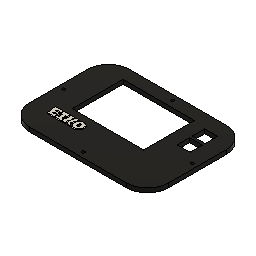
top plate (Autodesk Fusion 360 design; units mm, degrees)
part number: 2026-08-25-02-54-07-841
Autodesk Fusion 360 part; units mm, degrees
note: some values were not read from the file. Chosen so that the rebuilt part matches the saved one: which bodies a step acts on.
sketch "Sketch1" plane through (0, 0, 0) normal (0, 1, 0) x (1, 0, 0)
  line L0 (-1.5154, 62.1887) -> (-1.5154, -12.2213)
  line L1 (-112.7654, -12.2213) -> (-112.7654, 62.1887)
  line L2 (-112.7654, 62.1887) -> (-1.5154, 62.1887)
  line L3 (-1.5154, -12.2213) -> (-112.7654, -12.2213)
  line L4 (-122.7654, 72.1887) -> (8.4846, 72.1887)
  line L5 (-122.7654, -22.2213) -> (-122.7654, 72.1887)
  line L6 (8.4846, 72.1887) -> (8.4846, -22.2213)
  line L7 (8.4846, -22.2213) -> (-122.7654, -22.2213)
  circle A0 centre (-117.7654, 24.9837) radius 1.35
  circle A1 centre (-57.1404, 67.1887) radius 1.35
  circle A2 centre (3.4846, 24.9837) radius 1.35
  circle A3 centre (-57.1404, -17.2213) radius 1.35
sketch "Sketch2" plane through (0, 0, 0) normal (0, 1, 0) x (1, 0, 0)
  line L0 (-106.5854, 60.9687) -> (-21.5854, 60.9687)
  line L1 (-21.5854, 60.9687) -> (-21.5854, 12.9687)
  line L2 (-21.5854, 12.9687) -> (-106.5854, 12.9687)
  line L3 (-106.5854, 12.9687) -> (-106.5854, 60.9687)
  line L4 (-106.5854, 60.9687) -> (-21.5854, 60.9687)
  line L5 (-21.5854, 60.9687) -> (-21.5854, 12.9687)
  line L6 (-21.5854, 12.9687) -> (-106.5854, 12.9687)
  line L7 (-106.5854, 12.9687) -> (-106.5854, 60.9687)
  line L8 (-18.6954, 59) -> (-6.4954, 59)
  line L9 (-6.4954, 59) -> (-6.4954, 47.3)
  line L10 (-6.4954, 47.3) -> (-18.6954, 47.3)
  line L11 (-18.6954, 47.3) -> (-18.6954, 59)
  line L12 (-18.6954, 44.63) -> (-6.4954, 44.63)
  line L13 (-6.4954, 44.63) -> (-6.4954, 32.93)
  line L14 (-6.4954, 32.93) -> (-18.6954, 32.93)
  line L15 (-18.6954, 32.93) -> (-18.6954, 44.63)
  line L16 (-97.8354, 60.9687) -> (-30.3354, 60.9687)
  line L17 (-30.3354, 60.9687) -> (-30.3354, 12.9687)
  line L18 (-30.3354, 12.9687) -> (-97.8354, 12.9687)
  line L19 (-97.8354, 12.9687) -> (-97.8354, 60.9687)
  dimension "d5" = 85
  dimension "d6" = 48
  dimension "d11" = 12.2
  dimension "d12" = 11.7
  dimension "d13" = 2.89
  dimension "d14" = 12.2
  dimension "d15" = 11.7
  dimension "d16" = 2.67
  dimension "d17" = 2.89
  dimension "d28" = 67.5
  dimension "d29" = 8.75
  constraint horizontal L0
  constraint vertical L1
  constraint horizontal L2
  constraint vertical L3
  constraint horizontal L4
  constraint vertical L5
  constraint horizontal L6
  constraint vertical L7
  constraint horizontal L8
  constraint vertical L9
  constraint horizontal L10
  constraint vertical L11
  constraint horizontal L12
  constraint vertical L13
  constraint horizontal L14
  constraint vertical L15
  constraint horizontal L16
  constraint vertical L17
  constraint horizontal L18
  constraint vertical L19
  constraint coincident L4 L16.start
  measures "d5" distance of L0.start L0.end
  measures "d6" distance of L0 L2
  measures "d11" distance of L8.start L8.end
  measures "d12" distance of L8.start L10.end
  measures "d13" distance of L5 L11
  measures "d14" distance of L12.start L12.end
  measures "d15" distance of L12.start L14.end
  measures "d16" distance of L10 L12
  measures "d17" distance of L5 L15
  measures "d28" distance of L16.start L16.end
  measures "d29" distance of L7 L19
extrude "Extrude1" add sketch "Sketch1" along normal blind 4 contours L0 L1 L2 L3 | L4 L5 L6 L7 makes body 1
sketch "Sketch3" plane through (0, 4, 0) normal (0, 1, 0) x (-1, 0, 0)
  circle A0 centre (117.7654, -24.9837) radius 1.35
  circle A1 centre (57.1404, 17.2213) radius 1.35
  circle A2 centre (-3.4846, -24.9837) radius 1.35
  circle A3 centre (57.1404, -67.1887) radius 1.35
  line L0 (-8.4846, 22.2213) -> (-8.4846, -72.1887)
  line L1 (-8.4846, -72.1887) -> (122.7654, -72.1887)
  line L2 (122.7654, -72.1887) -> (122.7654, 22.2213)
  line L3 (122.7654, 22.2213) -> (-8.4846, 22.2213)
extrude "Extrude2" cut sketch "Sketch2" along normal blind 10 bodies 1
fillet "Fillet1" radius 20 4 edges at (-122.7654, 2, 22.2213) (8.4846, 2, 22.2213) (8.4846, 2, -72.1887) (-122.7654, 2, -72.1887) on bodies 1
sketch "Sketch4" plane through (0, 4, 0) normal (0, 1, 0) x (-1, 0, 0)
sketch "Sketch5" plane through (0, 4, 0) normal (0, 1, 0) x (-1, 0, 0)
  line L0 (99.062, -5.8308) -> (106.6622, -5.8308)
  line L1 (106.6622, -5.8308) -> (105.2136, 2.8806)
  line L2 (105.2136, 2.8806) -> (98.804, 2.9004)
  line L3 (98.804, 2.9004) -> (98.804, -0.1357)
  line L4 (98.804, -0.1357) -> (102.8919, 0.8168)
  line L5 (102.8919, 0.8168) -> (102.8919, -0.5325)
  line L6 (102.8919, -0.5325) -> (98.9231, -0.5325)
  line L7 (98.9231, -0.5325) -> (99.062, -2.6955)
  line L8 (99.062, -2.6955) -> (102.8919, -2.4177)
  line L9 (102.8919, -2.4177) -> (102.6934, -3.8068)
  line L10 (102.6934, -3.8068) -> (98.804, -3.1519)
  line L11 (98.804, -3.1519) -> (99.062, -5.8308)
  line L12 (98.2484, 0.539) -> (98.2484, 2.9798)
  line L13 (98.2484, 2.9798) -> (92.5334, 2.8806)
  line L14 (92.5334, 2.8806) -> (92.6922, 0.539)
  line L15 (92.6922, 0.539) -> (94.0217, 0.4795)
  line L16 (94.0217, 0.4795) -> (94.0217, -2.9535)
  line L17 (94.0217, -2.9535) -> (92.5533, -3.1916)
  line L18 (92.5533, -3.1916) -> (92.6922, -6.0491)
  line L19 (92.6922, -6.0491) -> (98.4667, -6.0491)
  line L20 (98.4667, -6.0491) -> (98.4667, -2.5963)
  line L21 (98.4667, -2.5963) -> (96.8792, -2.8543)
  line L22 (96.8792, -2.8543) -> (96.7006, 0.539)
  line L23 (96.7006, 0.539) -> (98.2484, 0.539)
  line L24 (91.819, -6.0094) -> (91.5809, -0.5921)
  line L25 (91.5809, -0.5921) -> (92.0373, -0.5921)
  line L26 (92.0373, -0.5921) -> (92.0373, 2.7417)
  line L27 (92.0373, 2.7417) -> (89.0806, 2.7417)
  line L28 (89.0806, 2.7417) -> (89.0806, -0.5921)
  line L29 (89.0806, -0.5921) -> (86.739, 2.7417)
  line L30 (86.739, 2.7417) -> (84.199, 2.7417)
  line L31 (84.199, 2.7417) -> (86.4612, -0.5921)
  line L32 (86.4612, -0.5921) -> (85.8262, -0.5921)
  line L33 (85.8262, -0.5921) -> (83.6633, -6.0094)
  line L34 (83.6633, -6.0094) -> (87.1161, -6.0094)
  line L35 (87.1161, -6.0094) -> (88.2472, -0.7905)
  line L36 (88.2472, -0.7905) -> (88.2472, -5.8308)
  line L37 (88.2472, -5.8308) -> (91.819, -6.0094)
  line L38 (78.7222, 2.7417) -> (82.4726, 2.7417)
  line L39 (82.4726, 2.7417) -> (84.199, -0.473)
  line L40 (84.199, -0.473) -> (84.199, -3.7671)
  line L41 (84.199, -3.7671) -> (82.4726, -5.9697)
  line L42 (82.4726, -5.9697) -> (78.7222, -5.9697)
  line L43 (78.7222, -5.9697) -> (76.0234, -4.4418)
  line L44 (76.0234, -4.4418) -> (76.0234, 0.162)
  line L45 (76.0234, 0.162) -> (78.7222, 2.7417)
sketch "Sketch6" plane through (0, 4, 0) normal (0, 1, 0) x (-1, 0, 0)
  arc A0 (102.7654, -72.1887) -> (122.7654, -52.1887) centre (102.7654, -52.1887) ccw
  line L0 (122.7654, -52.1887) -> (122.7654, 2.2213)
  arc A1 (122.7654, 2.2213) -> (102.7654, 22.2213) centre (102.7654, 2.2213) ccw
  line L1 (102.7654, 22.2213) -> (11.5154, 22.2213)
  arc A2 (11.5154, 22.2213) -> (-8.4846, 2.2213) centre (11.5154, 2.2213) ccw
  line L2 (-8.4846, 2.2213) -> (-8.4846, -52.1887)
  arc A3 (-8.4846, -52.1887) -> (11.5154, -72.1887) centre (11.5154, -52.1887) ccw
  line L3 (11.5154, -72.1887) -> (102.7654, -72.1887)
  circle A4 centre (57.1404, -67.1887) radius 1.35
  circle A5 centre (-3.4846, -24.9837) radius 1.35
  circle A6 centre (57.1404, 17.2213) radius 1.35
  circle A7 centre (117.7654, -24.9837) radius 1.35
  line L4 (18.6954, -32.93) -> (18.6954, -44.63)
  line L5 (18.6954, -44.63) -> (6.4954, -44.63)
  line L6 (6.4954, -44.63) -> (6.4954, -32.93)
  line L7 (6.4954, -32.93) -> (18.6954, -32.93)
  line L8 (18.6954, -47.3) -> (18.6954, -59)
  line L9 (18.6954, -59) -> (6.4954, -59)
  line L10 (6.4954, -59) -> (6.4954, -47.3)
  line L11 (6.4954, -47.3) -> (18.6954, -47.3)
  line L12 (106.5854, -12.9687) -> (106.5854, -60.9687)
  line L13 (106.5854, -60.9687) -> (21.5854, -60.9687)
  line L14 (21.5854, -60.9687) -> (21.5854, -12.9687)
  line L15 (21.5854, -12.9687) -> (106.5854, -12.9687)
  spline S0 degree 5 poles (81.2674, -1.8727) (81.2639, -1.9898) (81.2506, -2.2237) (81.212, -2.5678) (81.1218, -2.9909) (80.9363, -3.4119) (80.6735, -3.686) (80.3388, -3.7866) (79.9555, -3.7035) (79.5706, -3.4464) (79.2413, -3.0405) (79.0234, -2.5232) (78.9592, -1.9416) (79.0643, -1.349) (79.3168, -0.8028) (79.6717, -0.3579) (80.0714, -0.0622) (80.4582, 0.05) (80.7853, -0.0367) (81.0302, -0.3115) (81.1894, -0.7419) (81.2539, -1.1732) (81.2717, -1.5208) (81.2709, -1.7555) (81.2674, -1.8727) knots 0 0 0 0 0 0 0.05 0.1 0.15 0.2 0.25 0.3 0.35 0.4 0.45 0.5 0.55 0.6 0.65 0.7 0.75 0.8 0.85 0.9 0.95 1 1 1 1 1 1
  point P0 (80.3684, -3.7386)
  point P1 (79, -2)
  point P2 (80.5, 0)
extrude "Extrude3" add sketch "Sketch5" along normal blind 1 separate body makes body 2 at (-89.7156, 4, -4.1441) makes body 3 at (-96.0127, 4, -4.9842) makes body 4 at (-79.6482, 4, -2.0936) makes body 5 at (-104.9225, 4, -1.1609)
extrude "Extrude4" cut sketch "Sketch6" along normal blind 3 contours S0 bodies 4
extrude "Extrude5" add sketch "Sketch2" along normal blind 4 contours L0 L2 L3 L4 L6 L7 L19 bodies 1
extrude "Extrude6" add sketch "Sketch2" along normal blind 4 contours L0 L1 L2 L4 L5 L6 L17 bodies 1
